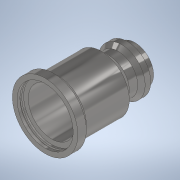
# Autodesk Inventor part: Для регулировки 3
Saved by Autodesk Inventor 2021 (Build 250183000, 183)
## iProperties
Created: 2020-12-19
Part Number: Для регулировки 3
Material: Сталь, высокопрочная, низколегированная
Document SubType Name: Modeling
Designer: Тимоха
Mass: 415.341 g
Surface Area: 236.434 cm^2
Volume: 52.9097 cm^3
Density: 7.85 g/cm^3
Appearance: Сталь — полированная
Author: Тимоха
Autodesk Inventor part; units mm, degrees
ref_plane "YZ Plane" through (0, 0, 0) normal (1, 0, 0) x (0, 1, 0)
ref_plane "XZ Plane" through (0, 0, 0) normal (0, 1, 0) x (-1, 0, 0)
ref_plane "XY Plane" through (0, 0, 0) normal (0, 0, 1) x (1, 0, 0)
sketch "Эскиз1" plane through (0, 0, 0) normal (0, 0, 1) x (1, 0, 0)
  circle A0 centre (0, 0) radius 17.5
  circle A1 centre (0, 0) radius 25
  dimension "d0" = 35
  dimension "d1" = 50
  constraints: 2 centre point, 2 coincident
  measures "d0" diameter of A0
  measures "d1" diameter of A1
extrude "Выдавливание1" add sketch "Эскиз1" along normal blind 10
sketch "Эскиз2" plane through (0, 0, 10) normal (0, 0, 1) x (1, 0, 0)
  circle A0 centre (0, 0) radius 17.5 projected
  circle A1 centre (0, 0) radius 21
  dimension "d4" = 42
  constraints: 1 centre point, 1 coincident
  measures "d4" diameter of A1
extrude "Выдавливание2" add sketch "Эскиз2" along normal blind 18
sketch "Эскиз5" plane through (0, 0, 28) normal (0, 0, 1) x (1, 0, 0)
  circle A0 centre (0, 0) radius 21 projected
  circle A1 centre (0, 0) radius 17.5 projected
  circle A2 centre (0, 0) radius 30
  dimension "d20" = 60
  constraints: 1 centre point, 1 coincident
  measures "d20" diameter of A2
extrude "Выдавливание5" add sketch "Эскиз5" along normal blind 1 contours A0 | A2
sketch "Эскиз3" plane through (0, 0, 29) normal (0, 0, 1) x (1, 0, 0)
  circle A0 centre (0, 0) radius 21 projected
  circle A1 centre (0, 0) radius 30
  circle A2 centre (0, 0) radius 25
  dimension "d7" = 60
  dimension "d13" = 50
  constraints: 2 centre point, 2 coincident
  measures "d7" diameter of A1
  measures "d13" diameter of A2
extrude "Выдавливание3" add sketch "Эскиз3" along normal blind 50 contours A1
chamfer "Фаска1" distance 4 angle 45 1 edges at (-25, 0, 10)
sketch "Эскиз4" plane through (0, 0, 0) normal (0, 0, -1) x (-1, 0, 0)
  circle A0 centre (0, 0) radius 17.5 projected
  circle A1 centre (0, 0) radius 20
  dimension "d17" = 40
  constraints: 1 centre point, 1 coincident
  measures "d17" diameter of A1
extrude "Выдавливание4" add sketch "Эскиз4" along normal blind 8
chamfer "Фаска3" distance 9 angle 45 1 edges at (-21, 0, 28)
sketch "Эскиз6" plane through (0, 0, 79) normal (0, 0, 1) x (1, 0, 0)
  circle A0 centre (0, 0) radius 30 projected
  circle A1 centre (0, 0) radius 25 projected
  circle A2 centre (0, 0) radius 35
  dimension "d26" = 70
  constraints: 1 centre point, 1 coincident
  measures "d26" diameter of A2
extrude "Выдавливание6" add sketch "Эскиз6" along normal blind 2 contours A0 | A2
sketch "Эскиз7" plane through (0, 0, 81) normal (0, 0, 1) x (1, 0, 0)
  circle A0 centre (0, 0) radius 35 projected
  circle A1 centre (0, 0) radius 30
  dimension "d29" = 60
  constraints: 1 centre point, 1 coincident
  measures "d29" diameter of A1
extrude "Выдавливание7" add sketch "Эскиз7" along normal blind 7
chamfer "Фаска4" distance 5 angle 45 1 edges at (-30, 0, 79)
sketch "Эскиз8" plane through (0, 0, 0) normal (0, 1, 0) x (-1, 0, 0)
  line L0 (30, 81) -> (-30, 81) projected
  line L1 (30, 81) -> (30, 83)
  line L2 (30, 88) -> (30, 81) projected
  line L3 (30, 83) -> (32, 83)
  line L4 (32, 83) -> (32, 85)
  line L5 (32, 85) -> (30, 85)
  line L6 (0, -27.2) -> (0, 107.2) projected
  point P0 (0, 0)
  dimension "d35" = 2
  dimension "d36" = 2
  dimension "d37" = 2
  constraints: 8 end point, 3 perpendicular, 2 point on line
  measures "d35" distance of L0.start L1.end
  measures "d36" distance of L1.end L3.end
  measures "d37" distance of L3.end L4.end
revolve "Вращение1" cut sketch "Эскиз8" angle 360 about axis through (0, 0, -10) along (0, 0, 1)
